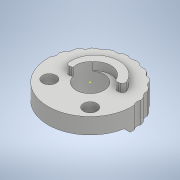
# Autodesk Inventor part: knob_bearing
Saved by Autodesk Inventor 2021 (Build 250183000, 183)
## iProperties
Created: 2017-06-22
Part Number: knob_bearing
Material: Generic
Document SubType Name: Modeling
Designer: theso
Density: 1 g/cm^3
Appearance: Default
Author: theso
Autodesk Inventor part; units mm, degrees
ref_plane "YZ Plane" through (0, 0, 0) normal (1, 0, 0) x (0, 1, 0)
ref_plane "XZ Plane" through (0, 0, 0) normal (0, 1, 0) x (-1, 0, 0)
ref_plane "XY Plane" through (0, 0, 0) normal (0, 0, 1) x (1, 0, 0)
sketch "Sketch1" plane through (0, 0, 0) normal (0, 0, 1) x (1, 0, 0)
  circle A0 centre (0, 0) radius 15.75
  dimension "d0" = 31.5
  constraints: 1 centre point, 1 coincident
  measures "d0" diameter of A0
extrude "Extrusion1" add sketch "Sketch1" along normal blind 4
sketch "Sketch2" plane through (0, 0, 4) normal (0, 0, 1) x (1, 0, 0)
  circle A0 centre (0, 0) radius 15.75 projected
  arc A1 (15.5107, -2.735) -> (-15.5107, -2.735) centre (0, 0) ccw
  line L0 (0, 0) -> (-15.5107, -2.735) construction
  line L1 (0, 0) -> (15.75, 0) construction
  line L2 (0, 0) -> (15.5107, -2.735) construction
  arc A2 (12.8025, -2.2574) -> (-12.8025, -2.2574) centre (0, 0) ccw
  line L3 (0, 0) -> (-12.8025, -2.2574) construction
  line L4 (0, 0) -> (13, 0) construction
  line L5 (0, 0) -> (12.8025, -2.2574) construction
  line L6 (-12.8025, -2.2574) -> (-15.5107, -2.735)
  line L7 (12.8025, -2.2574) -> (15.5107, -2.735)
  dimension "d3" = 170
  dimension "d4" = 160
  dimension "d5" = 13
  dimension "d6" = 170
  dimension "d7" = 160
  constraints: 16 end point, 5 point on circle, 2 centre point, 2 coincident, 2 equal length, 2 horizontal
  measures "d3" angle of L0 L1
  measures "d4" angle of L0 L2
  measures "d5" radius of A2
  measures "d6" angle of L3 L4
  measures "d7" angle of L3 L5
extrude "Extrusion2" add sketch "Sketch2" along normal blind 2 and the other way blind 6 contours A0 L7 A2 L6 picked at (-14.6775, -1.3371)
sketch "Sketch3" plane through (0, 0, 6) normal (0, 0, 1) x (1, 0, 0)
  arc A0 (15.5107, -2.735) -> (-15.5107, -2.735) centre (0, 0) ccw projected
  line L0 (0, 15.75) -> (0, 17.75)
  circle A1 centre (0, 17.75) radius 2.5
  line L1 (-4.4373, 15.112) -> (-5.0008, 17.031)
  circle A2 centre (-5.0008, 17.031) radius 2.5
  line L2 (-8.5151, 13.2497) -> (-9.5964, 14.9323)
  circle A3 centre (-9.5964, 14.9323) radius 2.5
  line L3 (-11.9031, 10.3141) -> (-13.4146, 11.6238)
  circle A4 centre (-13.4146, 11.6238) radius 2.5
  line L4 (-14.3267, 6.5428) -> (-16.146, 7.3736)
  circle A5 centre (-16.146, 7.3736) radius 2.5
  line L5 (-15.5897, 2.2415) -> (-17.5693, 2.5261)
  circle A6 centre (-17.5693, 2.5261) radius 2.5
  line L6 (-15.5897, -2.2415) -> (-17.5693, -2.5261)
  circle A7 centre (-17.5693, -2.5261) radius 2.5
  line L7 (-14.3267, -6.5428) -> (-16.146, -7.3736)
  circle A8 centre (-16.146, -7.3736) radius 2.5
  line L8 (-11.9031, -10.3141) -> (-13.4146, -11.6238)
  circle A9 centre (-13.4146, -11.6238) radius 2.5
  line L9 (-8.5151, -13.2497) -> (-9.5964, -14.9323)
  circle A10 centre (-9.5964, -14.9323) radius 2.5
  line L10 (-4.4373, -15.112) -> (-5.0008, -17.031)
  circle A11 centre (-5.0008, -17.031) radius 2.5
  line L11 (0, -15.75) -> (0, -17.75)
  circle A12 centre (0, -17.75) radius 2.5
  line L12 (4.4373, -15.112) -> (5.0008, -17.031)
  circle A13 centre (5.0008, -17.031) radius 2.5
  line L13 (8.5151, -13.2497) -> (9.5964, -14.9323)
  circle A14 centre (9.5964, -14.9323) radius 2.5
  line L14 (11.9031, -10.3141) -> (13.4146, -11.6238)
  circle A15 centre (13.4146, -11.6238) radius 2.5
  line L15 (14.3267, -6.5428) -> (16.146, -7.3736)
  circle A16 centre (16.146, -7.3736) radius 2.5
  line L16 (15.5897, -2.2415) -> (17.5693, -2.5261)
  circle A17 centre (17.5693, -2.5261) radius 2.5
  line L17 (15.5897, 2.2415) -> (17.5693, 2.5261)
  circle A18 centre (17.5693, 2.5261) radius 2.5
  line L18 (14.3267, 6.5428) -> (16.146, 7.3736)
  circle A19 centre (16.146, 7.3736) radius 2.5
  line L19 (11.9031, 10.3141) -> (13.4146, 11.6238)
  circle A20 centre (13.4146, 11.6238) radius 2.5
  line L20 (8.5151, 13.2497) -> (9.5964, 14.9323)
  circle A21 centre (9.5964, 14.9323) radius 2.5
  line L21 (4.4373, 15.112) -> (5.0008, 17.031)
  circle A22 centre (5.0008, 17.031) radius 2.5
  dimension "d12" = 2
  dimension "d13" = 5
  dimension "d16" = 360
  constraints: 44 end point, 22 centre point, 22 coincident, 1 point on circle, 1 vertical, 111 other
  measures "d12" distance of L0.start L0.end
  measures "d13" diameter of A1
extrude "Extrusion3" cut sketch "Sketch3" against normal blind 9.25 contours A18 A0 | A0 A18 | A19 A0 | A0 A19 | A20 A0 | A0 A20 | A21 A0 | A0 A21 | A22 A0 | A0 A22 | A1 A0 | A0 A1 | A2 A0 | A0 A2 | A3 A0 | A0 A3 | A4 A0 | A0 A4 | A5 A0 | A0 A5 | A6 A0 | A0 A6
sketch "Sketch4" plane through (0, 0, 4) normal (0, 0, 1) x (1, 0, 0)
  circle A0 centre (0, 0) radius 3.05
  dimension "d20" = 6.1
  constraints: 1 centre point, 1 coincident
  measures "d20" diameter of A0
extrude "Extrusion4" cut sketch "Sketch4" along normal blind 9.25 and the other way blind 8.875
chamfer "Chamfer1" distance 2 angle 45 4 edges at (-14.1566, -2.4962, 6) (-14.1566, -2.4962, -2) (14.1566, -2.4962, 6) (14.1566, -2.4962, -2)
sketch "Sketch5" plane through (0, 0, 4) normal (0, 0, 1) x (1, 0, 0)
  line L0 (0, 0) -> (12.557, 3.3646)
  arc A0 (12.9974, -0.2609) -> (-12.9974, -0.2609) centre (0, 0) ccw projected
  line L1 (0, 0) -> (13, 0) construction
  line L2 (0, 0) -> (2.8978, 0.7765)
  circle A1 centre (0, 0) radius 3.05 projected
  line L3 (0, 0) -> (1.4489, 0.3882)
  arc A2 (7.2444, 1.9411) -> (-4.3467, -1.1647) centre (1.4489, 0.3882) ccw
  line L4 (1.4489, 0.3882) -> (7.2444, 1.9411) construction
  line L5 (1.4489, 0.3882) -> (-4.3467, -1.1647) construction
  arc A3 (10.1422, 2.7176) -> (-7.2444, -1.9411) centre (1.4489, 0.3882) ccw
  line L6 (-7.2444, -1.9411) -> (-4.3467, -1.1647)
  line L7 (7.2444, 1.9411) -> (10.1422, 2.7176)
  dimension "d26" = 15
  dimension "d33" = 1.5
  dimension "d34" = 6
  dimension "d35" = 180
  dimension "d36" = 9
  constraints: 16 end point, 6 point on circle, 5 point on line, 2 centre point, 2 coincident, 1 equal length, 1 horizontal, 1 midpoint, 1 other
  measures "d26" angle of L1 L0
  measures "d33" distance of L3.start L3.end
  measures "d34" radius of A2
  measures "d35" angle of L4 L5
  measures "d36" radius of A3
extrude "Extrusion5" add sketch "Sketch5" along normal blind 5 contours A2 L6 A3 L0
sketch "Sketch6" plane through (0, 0, 0) normal (0, 0, -1) x (-1, 0, 0)
  circle A0 centre (0, 0) radius 3.5
  circle A1 centre (0, 0) radius 7
  dimension "d38" = 14
  constraints: 2 centre point, 2 coincident
  measures "d38" diameter of A1
extrude "Extrusion6" add sketch "Sketch6" along normal blind 2
sketch "Sketch7" plane through (0, 0, 4) normal (0, 0, 1) x (1, 0, 0)
  arc A0 (-15.7278, 0.8353) -> (-15.7325, -0.7432) centre (0, 0) ccw projected
  arc A1 (15.7325, -0.7432) -> (15.7278, 0.8353) centre (0, 0) ccw projected
  arc A2 (-15.7278, 0.8353) -> (15.7325, -0.7432) centre (0, 0) ccw
  arc A3 (12.9974, -0.2609) -> (-12.9974, -0.2609) centre (0, 0) ccw projected
  arc A4 (-13, 0) -> (13, 0) centre (0, 0) ccw
  line L0 (0, 0) -> (13, 0) construction
  line L1 (0, 0) -> (-13, 0) construction
  line L2 (-15.7278, 0.8353) -> (-13, 0)
  line L3 (13, 0) -> (15.7278, 0.8353)
  dimension "d41" = 13
  dimension "d42" = 180
  constraints: 8 end point, 6 point on circle, 2 centre point, 2 coincident
  measures "d41" radius of A4
  measures "d42" angle of L1 L0
extrude "Extrusion7" add sketch "Sketch7" along normal blind 2 contours L2 A3 A4 L3 A1 A2 A0
sketch "Sketch12" plane through (0, 0, 4) normal (0, 0, 1) x (1, 0, 0)
  circle A0 centre (0, 0) radius 13
  constraints: 1 centre point, 1 coincident
extrude "Extrusion11" add sketch "Sketch12" along normal blind 2
sketch "Sketch8" plane through (0, 0, 0) normal (0, 0, -1) x (-1, 0, 0)
  arc A0 (-6.62, -8.785) -> (7.502, -8.0449) centre (0, 0) ccw
  line L0 (0, 0) -> (-6.62, -8.785) construction
  line L1 (0, 0) -> (11, 0) construction
  line L2 (0, 0) -> (7.502, -8.0449) construction
  circle A1 centre (-6.62, -8.785) radius 2.5
  circle A2 centre (7.502, -8.0449) radius 2.5
  dimension "d45" = 11
  dimension "d46" = 127
  dimension "d47" = 80
  dimension "d48" = 5
  dimension "d49" = 5
  constraints: 6 end point, 3 centre point, 3 coincident, 2 point on circle, 1 equal length, 1 horizontal
  measures "d45" radius of A0
  measures "d46" angle of L0 L1
  measures "d47" angle of L0 L2
  measures "d48" diameter of A1
  measures "d49" diameter of A2
extrude "Extrusion8" [suppressed]
sketch "Sketch13" plane through (0, 0, 6) normal (0, 0, 1) x (1, 0, 0)
  circle A0 centre (0, 0) radius 3.15
  dimension "d72" = 6.3
  constraints: 1 centre point, 1 coincident
  measures "d72" diameter of A0
extrude "Extrusion12" cut sketch "Sketch13" against normal blind 10.25
sketch "Sketch14" plane through (0, 0, 6) normal (0, 0, 1) x (1, 0, 0)
  point P0 (0, 0)
sketch "Sketch15" plane through (0, 0, 6) normal (0, 0, 1) x (1, 0, 0)
  arc A0 (-8.6212, -6.6525) -> (8.1676, -8.1213) centre (0.3894, -0.3431) ccw
  line L0 (0.3894, -0.3431) -> (-8.6212, -6.6525) construction
  line L1 (0.3894, -0.3431) -> (11.3894, -0.3431) construction
  line L2 (0.3894, -0.3431) -> (8.1676, -8.1213) construction
  circle A1 centre (-8.6212, -6.6525) radius 2.55
  circle A2 centre (8.1676, -8.1213) radius 2.55
  point P0 (0, 0)
  dimension "d73" = 11
  dimension "d74" = 145
  dimension "d75" = 100
  dimension "d76" = 5.1
  dimension "d77" = 5.1
  constraints: 6 end point, 3 centre point, 3 coincident, 2 point on circle, 1 equal length, 1 horizontal
  measures "d73" radius of A0
  measures "d74" angle of L0 L1
  measures "d75" angle of L0 L2
  measures "d76" diameter of A1
  measures "d77" diameter of A2
extrude "Extrusion13" cut sketch "Sketch15" against normal blind 5
fillet "Fillet6" radius 1.2 4 edges at (-7.2444, -1.9411, 7.5) (-4.3467, -1.1647, 7.5) (7.2444, 1.9411, 7.5) (10.1422, 2.7176, 7.5)
sketch "Sketch16" plane through (-8.6212, -6.6525, 1) normal (0, 0, 1) x (1, 0, 0)
  circle A0 centre (0, 0) radius 1
  circle A1 centre (16.7888, -1.4688) radius 2.55 projected
  circle A2 centre (16.7888, -1.4688) radius 1
  point P0 (8.6212, 6.6525)
  dimension "d84" = 2
  dimension "d85" = 2
  constraints: 2 centre point, 1 coincident
  measures "d84" diameter of A0
  measures "d85" diameter of A2
extrude "Extrusion14" [suppressed]
sketch "Sketch18" plane through (0, 0, 6) normal (0, 0, 1) x (1, 0, 0)
  arc A0 (-1.4115, 15.6866) -> (-3.0651, 15.4489) centre (0, 0) ccw projected
  line L0 (-3.0651, 15.4489) -> (-2.0298, 19.3126)
  line L1 (-3.0651, 15.4489) -> (0.9349, 15.4489) construction
  arc A1 (3.0651, 15.4489) -> (1.4115, 15.6866) centre (0, 0) ccw projected
  arc A2 (3.0651, 15.4489) -> (5.7738, 14.6535) centre (5.0008, 17.031) ccw projected
  line L2 (3.0651, 15.4489) -> (2.0298, 19.3126)
  line L3 (3.0651, 15.4489) -> (7.0651, 15.4489) construction
  line L4 (2.0298, 19.3126) -> (-2.0298, 19.3126)
  arc A3 (-5.7738, 14.6535) -> (-3.0651, 15.4489) centre (-5.0008, 17.031) ccw projected
  line L5 (-3.0651, 15.4489) -> (0.0694, 13.9872)
  line L6 (-3.0651, 15.4489) -> (0.3935, 15.4489) construction
  line L7 (0.0694, 13.9872) -> (3.0651, 15.4489)
  dimension "d94" = 4
  dimension "d95" = 75
  dimension "d96" = 4
  dimension "d97" = 105
  dimension "d98" = 25
  constraints: 16 end point, 3 equal length, 3 horizontal, 1 other
  measures "d94" distance of L0.start L0.end
  measures "d95" angle of L1 L0
  measures "d96" distance of L2.start L2.end
  measures "d97" angle of L3 L2
  measures "d98" angle of L5 L6
extrude "Extrusion16" [suppressed]
fillet "Fillet11" [suppressed]
sketch "Sketch20" plane through (0, 0, 6) normal (0, 0, 1) x (1, 0, 0)
  line L0 (-0.1809, 19.5537) -> (0.1809, 19.5537) projected
  arc A0 (-0.1809, 19.5537) -> (-2.5957, 17.7007) centre (-0.1809, 17.0537) ccw projected
  arc A1 (2.5957, 17.7007) -> (0.1809, 19.5537) centre (0.1809, 17.0537) ccw projected
  line L1 (-2.8685, 16.6827) -> (-2.5957, 17.7007) projected
  line L2 (2.5957, 17.7007) -> (2.8685, 16.6827) projected
  line L3 (-1.1298, 16.2169) -> (-0.8571, 17.2348)
  arc A2 (-0.1809, 17.7537) -> (-0.8571, 17.2348) centre (-0.1809, 17.0537) ccw
  line L4 (-0.1809, 17.7537) -> (0.1809, 17.7537)
  arc A3 (0.8571, 17.2348) -> (0.1809, 17.7537) centre (0.1809, 17.0537) ccw
  line L5 (0.8571, 17.2348) -> (1.1298, 16.2169)
  line L6 (-1.1298, 16.2169) -> (-1.6475, 14.285)
  line L7 (-1.6475, 14.285) -> (1.6475, 14.285)
  line L8 (1.6475, 14.285) -> (1.1298, 16.2169)
  point P0 (0, 0)
  dimension "d112" = 1.8
  dimension "d113" = 2
  constraints: 12 end point, 4 point on circle, 2 centre point, 1 collinear, 1 horizontal, 4 other
  measures "d112" radial gap between concentric circles of A0 A2
  measures "d113" distance of L3.start L6.end
extrude "Extrusion18" [suppressed]
fillet "Fillet12" [suppressed]
sketch "Sketch21" plane through (0, 0, -2) normal (0, 0, -1) x (-1, 0, 0)
  circle A0 centre (0, 0) radius 5.25
  dimension "d114" = 10.5
  constraints: 1 centre point, 1 coincident
  measures "d114" diameter of A0
extrude "Extrusion19" cut sketch "Sketch21" against normal blind 12
body "Solid1"
